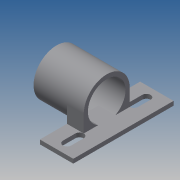
# Autodesk Inventor part: Bearing mount
Saved by Autodesk Inventor 2014 SP1 (Build 180222100, 222)
## iProperties
Created: 2014-02-01
Part Number: Bearing mount
Material: Generic
Document SubType Name: Modeling
Designer: Pradhan Alexander
Density: 1 g/cm^3
Appearance: Default
Author: Pradhan Alexander
Autodesk Inventor part; units mm, degrees
ref_plane "YZ Plane" through (0, 0, 0) normal (1, 0, 0) x (0, 1, 0)
ref_plane "XZ Plane" through (0, 0, 0) normal (0, 1, 0) x (-1, 0, 0)
ref_plane "XY Plane" through (0, 0, 0) normal (0, 0, 1) x (1, 0, 0)
sketch "Sketch1" plane through (0, 0, 0) normal (0, 1, 0) x (-1, 0, 0)
  line L0 (-3.4844, 10.1285) -> (-28.8844, 10.1285)
  line L1 (-28.8844, 10.1285) -> (-28.8844, -66.0715)
  line L2 (-28.8844, -66.0715) -> (-3.4844, -66.0715)
  line L3 (-3.4844, -66.0715) -> (-3.4844, 10.1285)
  dimension "d0" = 25.4
  dimension "d1" = 76.2
  constraints: 8 end point, 2 parallel, 1 horizontal, 1 perpendicular
  measures "d0" distance of L0.start L0.end
  measures "d1" distance of L2.end L0.start
extrude "Extrusion1" add sketch "Sketch1" against normal blind 3.175
sketch "Sketch7" plane through (3.4844, 0, -66.0715) normal (-1, 0, 0) x (0, 0, 1)
  line L0 (76.2, -3.175) -> (0, -3.175) projected
  circle A0 centre (38.1, 12.7254) radius 6.35
  circle A1 centre (38.1, 12.7254) radius 14.3002
  arc A2 (45.3498, -3.175) -> (30.8502, -3.175) centre (38.1, 12.7254) ccw
  dimension "d24" = 15.9004
  dimension "d25" = 12.7
  dimension "d26" = 28.6004
  dimension "d27" = 3.175
  constraints: 3 centre point, 2 coincident, 2 point on circle, 2 point on line
  measures "d24" distance from line of L0 A0.centre
  measures "d25" diameter of A0
  measures "d26" diameter of A1
  measures "d27" radial gap between concentric circles of A1 A2
extrude "Extrusion7" add sketch "Sketch7" along normal mid plane 25.4 contours L0 A2
sketch "Sketch8" plane through (16.1844, 0, -66.0715) normal (1, 0, 0) x (0, 0, -1)
  line L0 (-26.1231, 0) -> (-31.5762, 0) projected
  arc A0 (-26.1231, 0) -> (-50.0769, 0) centre (-38.1, 12.7254) ccw projected
  arc A1 (-30.8502, -3.175) -> (-45.3498, -3.175) centre (-38.1, 12.7254) ccw projected
  line L1 (-55.5752, 12.7254) -> (-55.5752, 0)
  line L2 (-50.0769, 0) -> (-76.2, 0) projected
  line L3 (-20.6248, 12.7254) -> (-20.6248, 0)
  line L4 (-76.2, 0) -> (0, 0) projected
  constraints: 4 end point, 4 point on circle, 4 tangent, 2 point on line, 1 parallel, 1 perpendicular
extrude "Extrusion8" add sketch "Sketch8" against normal blind 12.7 contours A0 L3 L4 | L2 L1 A0
sketch "Sketch10" plane through (0, 0, 0) normal (0, 1, 0) x (1, 0, 0)
  line L0 (28.8844, -10.1285) -> (28.8844, 66.0715) projected
  arc A0 (13.0094, -2.191) -> (19.3594, -2.191) centre (16.1844, -2.191) ccw
  arc A1 (19.3594, 7.334) -> (13.0094, 7.334) centre (16.1844, 7.334) ccw
  line L1 (13.0094, 7.334) -> (13.0094, -2.191)
  line L2 (19.3594, 7.334) -> (19.3594, -2.191)
  line L3 (19.3594, 2.5715) -> (20.4652, 2.5715)
  line L4 (28.8844, 27.9715) -> (23.8268, 27.9715)
  arc A2 (19.3594, 58.134) -> (13.0094, 58.134) centre (16.1844, 58.134) ccw
  arc A3 (13.0094, 48.609) -> (19.3594, 48.609) centre (16.1844, 48.609) ccw
  line L5 (13.0094, 58.134) -> (13.0094, 48.609)
  line L6 (19.3594, 48.609) -> (19.3594, 58.134)
  line L7 (19.3594, 53.3715) -> (21.2976, 53.3715)
  line L8 (16.1844, 61.309) -> (16.1844, 45.434)
  line L9 (16.1844, 10.509) -> (16.1844, -5.366)
  dimension "d42" = 12.7
  dimension "d43" = 6.35
  dimension "d44" = 6.35
  dimension "d45" = 25.4
  dimension "d46" = 6.35
  dimension "d47" = 6.35
  dimension "d48" = 12.7
  dimension "d49" = 25.4
  dimension "d52" = 15.875
  dimension "d53" = 15.875
  constraints: 18 end point, 12 point on circle, 7 tangent, 4 centre point, 3 midpoint, 2 perpendicular, 1 parallel
  measures "d42" distance from line of L0 A0.centre
  measures "d43" diameter of A1
  measures "d44" diameter of A0
  measures "d45" distance between parallel lines of L4 L3
  measures "d46" diameter of A3
  measures "d47" diameter of A2
  measures "d48" distance from line of L0 A2.centre
  measures "d49" distance between parallel lines of L4 L7
  measures "d52" distance of L8.start L8.end
  measures "d53" distance of L9.start L9.end
extrude "Extrusion10" cut sketch "Sketch10" against normal blind 25.4
sketch "Sketch11" plane through (-9.2156, 0, -66.0715) normal (-1, 0, 0) x (0, 0, 1)
  circle A0 centre (38.1, 12.7254) radius 14.3002 projected
  arc A1 (45.3498, -3.175) -> (30.8502, -3.175) centre (38.1, 12.7254) ccw projected
  line L0 (30.8502, -3.175) -> (45.3498, -3.175) projected
extrude "Extrusion11" add sketch "Sketch11" along normal blind 12.7
body "Solid1"
